Autodesk Fusion 360 part; units mm, degrees
note: some values were not read from the file. Chosen so that the rebuilt part matches the saved one: which bodies a step acts on; which face or edge a step refers to. Set by a fixed rule: which sketch regions a step uses.
(part 2 of 2)
component "hægra afturhjól (1)" placed x (0, 0, 1) y (0, 1, 0) z (-1, 0, 0) at (-213, -5, 24)
component "framvængur" placed x (1, 0, 0) y (0, 0.984808, -0.173648) z (0, 0.173648, 0.984808) at (-230, 70.5116, -31.8297)
component "framöxull" placed x (0.766044, -0.642788, 0) y (0, 0, -1) z (0.642788, 0.766044, 0) at (-136.0942, -118.4155, -700.9616)
component "Component''''" placed x (0.766044, -0.642788, 0) y (0, 0, -1) z (0.642788, 0.766044, 0) at (-135.9354, -54.9066, -5.8797)
component "Body hægri (1)" placed x (0, 0, -1) y (0, 1, 0) z (1, 0, 0) at (-92.4102, -20, 22.4102)
component "hægra afturhjól (2)" placed x (0, 0, 1) y (0, 1, 0) z (-1, 0, 0) at (-126, 0, -28)
component "hægri afturvængsfesting1 (1)" placed x (0, 0, -1) y (-0.108193, -0.99413, 0) z (-0.99413, 0.108193, 0) at (-33.855, -49.9073, 25.4102)
component "hægri afturvængsfesting 2 (1)" placed x (1, 0, 0) y (0, -0.99413, -0.108193) z (0, 0.108193, -0.99413) at (-53.5469, -48.7181, 34.4604)
component "hægri hliðaplata (1)" placed x (0, 0, 1) y (0, 1, 0) z (-1, 0, 0) at (-15.4308, -183.2827, 78.8671)
component "afturvængur efri (1)" placed x (1, 0, 0) y (0, -0.866025, 0.5) z (0, -0.5, -0.866025) at (-230.5488, -77.2458, 47.5251)
component "afturvængur neðri (1)" placed x (1, 0, 0) y (0, -1, 0) z (0, 0, -1) at (-229.9121, -78.3584, 42.4102)
component "hægra afturhjól (1) (1)" placed x (0, 0, 1) y (0, 1, 0) z (-1, 0, 0) at (-118, 0, -36)
component "hægri hliðaplata" placed x (0, 0, -1) y (0, 1, 0) z (1, 0, 0) at (-64.7874, -139.521, 22.3531)
component "hægri afturvængsfesting 2" placed x (1, 0, 0) y (0, 0.99413, 0.108193) z (0, -0.108193, 0.99413) at (-27.8042, -58.3906, -22.64)
component "hægri afturvængsfesting1" placed x (0, 0, -1) y (-0.108193, -0.99413, 0) z (-0.99413, 0.108193, 0) at (-24.3461, -150.6331, 10.4102)
component "hægra afturhjól" placed x (0, 0, -1) y (0, 1, 0) z (1, 0, 0) at (-227, 0, -10)
component "Body hægri" placed x (0, -0.000138, -1) y (0.000138, 1, -0.000138) z (1, -0.000138, 0) at (-181.56, -0.0012, -8.44)
equation "thickness = 3 mm"
equation "d2 = thickness"
equation "d5 = thickness"
equation "d7 = thickness"
equation "d15 = thickness"
equation "d24 = thickness"
equation "d31 = dekkouter"
equation "dekkinner = 6.75 mm"
equation "dekkouter = 35 mm"
equation "d35 = thickness / 2"
equation "d37 = dekkouter"
equation "d38 = thickness / 2"
equation "d39 = -thickness"
equation "d44 = ( 13 / 3 ) * 1 mm"
equation "d45 = ( 13 / 3 ) * 1 mm"
equation "d46 = thickness"
equation "d47 = ( 13 / 3 ) * 1 mm"
equation "d48 = thickness"
equation "d49 = ( 13 / 3 ) * 1 mm"
equation "d50 = -thickness"
equation "d55 = ( 13 / 3 ) * 1 mm"
equation "d56 = thickness"
equation "d57 = ( 13 / 3 ) * 1 mm"
equation "d58 = -thickness"
equation "d60 = ( 13 / 3 ) * 1 mm"
equation "d61 = thickness"
equation "d62 = ( 13 / 3 ) * 1 mm"
equation "d63 = thickness"
equation "d64 = ( 13 / 3 ) * 1 mm"
equation "d71 = ( 13 / 3 ) * 1 mm"
equation "d72 = thickness"
equation "d74 = -thickness"
equation "d80 = ( 13 / 3 ) * 1 mm"
equation "d81 = thickness"
equation "d88 = thickness"
equation "d91 = thickness"
equation "d92 = thickness"
equation "d94 = thickness"
equation "d95 = thickness"
equation "d98 = thickness"
equation "d103 = thickness"
equation "d105 = 3 mm + 18 mm"
equation "d106 = 3 mm + 18 mm"
equation "d107 = thickness"
equation "d111 = thickness"
equation "d114 = 30 mm - 5 mm"
equation "d117 = -thickness"
named bodies: "Body hægri", "framöxull", "hægra afturhjól", "hægri afturvængsfesting1", "hægri afturvængsfesting 2", "hægri hliðaplata", "framvængur", "afturvængur efri", "afturvængur neðri", "hægra afturhjól (1)", "Body hægri (1)", "hægra afturhjól (2)", "hægri afturvængsfesting1 (1)", "hægri afturvængsfesting 2 (1)", "hægri hliðaplata (1)", "framvængur (1)", "afturvængur efri (1)", "afturvængur neðri (1)", "hægra afturhjól (1) (1)"
